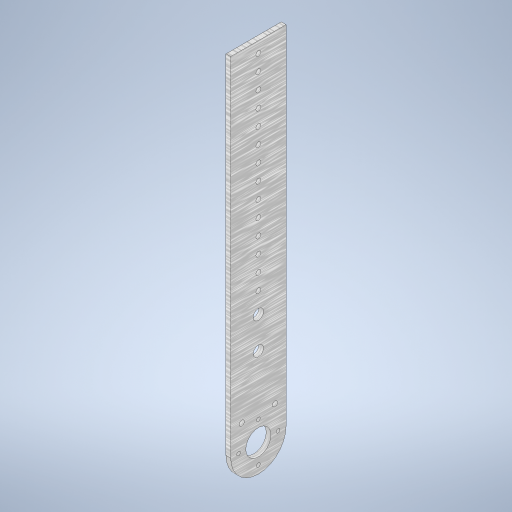
# Autodesk Inventor part: shoulder2_upper_plate_rigth
Saved by Autodesk Inventor 2024 (Build 280153000, 153)
## iProperties
Created: 2025-08-05
Part Number: shoulder2_upper_plate_rigth
Material: アルミニウム 5052
Document SubType Name: Modeling
Designer: HosodaLab2
Density: 2.68 g/cm^3
Appearance: サテン - ブラシ仕上げ 重厚
個数: 1
Author: HosodaLab2
Autodesk Inventor part; units mm, degrees
ref_plane "YZ Plane" through (0, 0, 0) normal (1, 0, 0) x (0, 1, 0)
ref_plane "XZ Plane" through (0, 0, 0) normal (0, 1, 0) x (-1, 0, 0)
ref_plane "XY Plane" through (0, 0, 0) normal (0, 0, 1) x (1, 0, 0)
sketch "スケッチ1" plane through (0, 0, 0) normal (0, 1, 0) x (-1, 0, 0)
  line L0 (0, 0) -> (-35, 0)
  line L1 (-35, 0) -> (-35, -220)
  line L2 (-35, -220) -> (0, -220)
  line L3 (0, -220) -> (0, 0)
  arc A0 (-35, -220) -> (0, -220) centre (-17.5, -220) ccw
  dimension "d0" = 35
  dimension "d1" = 220
  dimension "d2" = 17.5
  constraints: 8 end point, 2 parallel, 2 point on circle, 1 centre point, 1 horizontal, 1 perpendicular
  measures "d0" distance of L2.end L1.end
  measures "d1" distance of L1.end L0.end
  measures "d2" radius of A0
extrude "押し出し1" add sketch "スケッチ1" along normal blind 3
sketch "スケッチ2" plane through (0, 3, 0) normal (0, 1, 0) x (1, 0, 0)
  line L0 (0, 0) -> (35, 0) construction
  line L1 (17.5, 0) -> (17.5, 237.5) construction
  arc A0 (35, 220) -> (0, 220) centre (17.5, 220) ccw construction
  constraints: 2 end point, 1 coincident, 1 midpoint, 1 point on circle, 1 vertical
hole "穴1" at (17.5, 3, -220) direction (0, -1, 0) diameter 16 end through all
sketch "スケッチ3" plane through (0, 3, 0) normal (0, 1, 0) x (1, 0, 0)
  circle A0 centre (17.5, 220) radius 8 projected
  circle A1 centre (17.5, 220) radius 12.5
  point P0 (0, 0)
  point P1 (5, 220)
  point P2 (30, 220)
  point P3 (17.5, 232.5)
  point P4 (17.5, 207.5)
  dimension "d12" = 25
  constraints: 4 point on circle, 1 centre point, 1 coincident
  measures "d12" diameter of A1
hole "穴2" at (5, 3, -220) at (30, 3, -220) at (17.5, 3, -232.5) at (17.5, 3, -207.5) direction (0, -1, 0) diameter 2.459 end through all thread size "M3x0.5" class "6H" standard "ISO Metric profile"
sketch "スケッチ4" plane through (0, 3, 0) normal (0, 1, 0) x (1, 0, 0)
  line L0 (0, 0) -> (35, 0) construction
  line L1 (17.5, 0) -> (17.5, 237.5) construction
  arc A0 (35, 220) -> (0, 220) centre (17.5, 220) ccw construction
  circle A1 centre (17.5, 220) radius 8 projected
  point P0 (17.5, 137)
  point P1 (17.5, 127)
  point P2 (17.5, 117)
  point P3 (17.5, 107)
  point P4 (17.5, 97)
  point P5 (17.5, 87)
  point P6 (17.5, 77)
  point P7 (17.5, 67)
  point P8 (17.5, 57)
  point P9 (17.5, 47)
  point P10 (17.5, 37)
  point P11 (17.5, 27)
  point P12 (17.5, 17)
  point P13 (17.5, 7)
  dimension "d42" = 83
  dimension "d45" = 10
  constraints: 2 end point, 2 vertical, 1 midpoint, 1 point on circle, 13 other
  measures "d42" distance of A1.centre point (17.5, 137)
  measures "d45" distance of point (17.5, 137) point (17.5, 127)
hole "穴3" at (17.5, 3, -137) at (17.5, 3, -127) at (17.5, 3, -117) at (17.5, 3, -107) at (17.5, 3, -97) at (17.5, 3, -87) at (17.5, 3, -77) at (17.5, 3, -67) at (17.5, 3, -57) at (17.5, 3, -47) at (17.5, 3, -37) at (17.5, 3, -27) at (17.5, 3, -17) at (17.5, 3, -7) direction (0, -1, 0) diameter 3.2 end through all
sketch "スケッチ5" plane through (0, 3, 0) normal (0, 1, 0) x (1, 0, 0)
  line L0 (0, 0) -> (35, 0) construction
  line L1 (17.5, 0) -> (17.5, 237.5) construction
  arc A0 (35, 220) -> (0, 220) centre (17.5, 220) ccw construction
  circle A1 centre (17.5, 137) radius 1.6 construction
  point P0 (17.5, 150)
  point P1 (17.5, 170)
  dimension "d50" = 13
  dimension "d51" = 20
  constraints: 2 end point, 2 point on line, 1 midpoint, 1 point on circle, 1 vertical
  measures "d50" distance of point (17.5, 150) A1.centre
  measures "d51" distance of point (17.5, 170) point (17.5, 150)
hole "穴4" at (17.5, 3, -150) at (17.5, 3, -170) direction (0, -1, 0) diameter 6.6 end through all
sketch "スケッチ6" plane through (0, 3, 0) normal (0, 1, 0) x (1, 0, 0)
  line L0 (35, 0) -> (35, 220) projected
  line L1 (35, 204.2) -> (0, 204.2) construction
  line L2 (0, 220) -> (0, 0) projected
  circle A0 centre (17.5, 220) radius 8 projected
  line L3 (17.5, 220) -> (17.5, 204.2) construction
  point P0 (28, 204.2)
  point P1 (7, 204.2)
  dimension "d52" = 15.8
  dimension "d53" = 10.5
  dimension "d54" = 10.5
  constraints: 4 end point, 4 point on line, 1 horizontal, 1 midpoint
  measures "d52" distance from line of L3.start L1
  measures "d53" distance from line of L3 point (7, 204.2)
  measures "d54" distance of point (28, 204.2) L3.end
hole "穴5" at (28, 3, -204.2) at (7, 3, -204.2) direction (0, -1, 0) diameter 3.3 end through all
